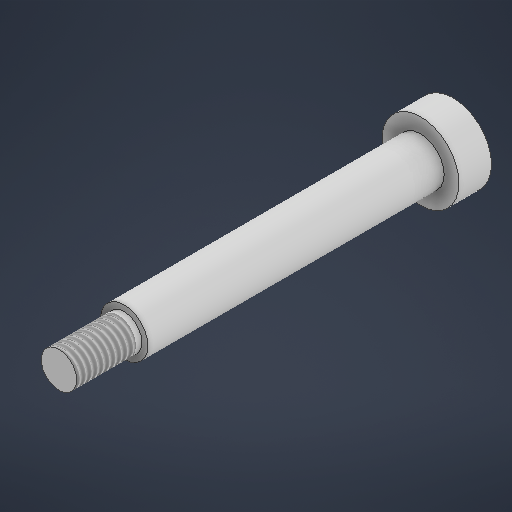
# Autodesk Inventor part: Shoulder bolt D8(M6) 60L
Saved by Autodesk Inventor 2025.3 (Build 293356000, 356)
## iProperties
Created: 2025-04-18
Part Number: Shoulder bolt D8(M6) 60L
Material: Generic
Document SubType Name: Modeling
Designer: Nelson
Density: 1 g/cm^3
Appearance: Default
Author: Nelson
Autodesk Inventor part; units mm, degrees
ref_plane "YZ Plane" through (0, 0, 0) normal (1, 0, 0) x (0, 1, 0)
ref_plane "XZ Plane" through (0, 0, 0) normal (0, 1, 0) x (-1, 0, 0)
ref_plane "XY Plane" through (0, 0, 0) normal (0, 0, 1) x (1, 0, 0)
sketch "Sketch1" plane through (0, 0, 0) normal (0, 0, 1) x (1, 0, 0)
  circle A0 centre (0, 0) radius 6.5
  circle A1 centre (0, 0) radius 2
  dimension "dk" = 13
  dimension "SS" = 4
  constraints: 2 centre point, 2 coincident
  measures "dk" diameter of A0
  measures "SS" diameter of A1
extrude "Extrusion1" add sketch "Sketch1" along normal blind 5.5 contours A0 | A1
sketch "Sketch2" plane through (0, 0, 5.5) normal (0, 0, 1) x (1, 0, 0)
  circle A0 centre (0, 0) radius 4
  dimension "D" = 8
  constraints: 1 centre point, 1 coincident
  measures "D" diameter of A0
extrude "Extrusion2" cut sketch "Sketch1" along normal blind 3 contours A1
extrude "Extrusion3" add sketch "Sketch2" along normal blind 50
sketch "Sketch3" plane through (0, 0, 55.5) normal (0, 0, 1) x (1, 0, 0)
  circle A0 centre (0, 0) radius 3
  dimension "dd" = 6
  constraints: 1 centre point, 1 coincident
  measures "dd" diameter of A0
extrude "Extrusion4" add sketch "Sketch3" along normal blind 11
thread "Thread1" size "M6x1" class "6g" standard "ISO Metric profile" length 10
body "Solid1"
